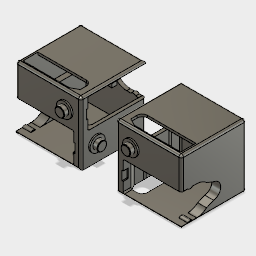
servo_assem_type2 (Autodesk Fusion 360 design; units mm, degrees)
Autodesk Fusion 360 part; units mm, degrees
sketch "スケッチ1" plane through (0, 0, 0) normal (0, 1, 0) x (1, 0, 0)
  line L0 (12.9, -12.9) -> (-12.9, -12.9)
  line L1 (-12.9, -12.9) -> (-12.9, 12.9)
  line L2 (-12.9, 12.9) -> (12.9, 12.9)
  line L3 (12.9, 12.9) -> (12.9, -12.9)
  line L4 (12.9, -12.9) -> (-12.9, 12.9) construction
  line L5 (-12.9, -12.9) -> (12.9, 12.9) construction
  line L6 (12.9, 12.9) -> (11.6, 12.9)
  line L7 (11.6, 12.9) -> (11.6, 11.4)
  line L8 (11.6, 11.4) -> (12.9, 11.4)
  line L9 (12.9, 11.4) -> (12.9, 12.9)
  line L10 (11.6, 11.4) -> (5.6, 11.4)
  line L11 (5.6, 11.4) -> (5.6, -9.858)
  line L12 (5.6, -9.858) -> (11.6, -9.858)
  line L13 (11.6, -9.858) -> (11.6, 11.4)
  line L14 (11.6, -9.858) -> (10.1, -9.858)
  line L15 (11.6, -9.858) -> (13.1, -9.858) construction
  line L16 (10.1, -9.858) -> (11.6, -7.0369)
  line L17 (10.1, -9.858) -> (13.2951, -9.858) construction
  dimension "d1" = 25.8
  dimension "d2" = 25.8
  dimension "d10" = 1.5
  dimension "d11" = 1.3
  dimension "d12" = 6
  dimension "d13" = 21.258
  dimension "d14" = 180
  dimension "d15" = 1.5
  dimension "d16" = 62
  constraint perpendicular L0 L1
  constraint parallel L0 L2
  constraint parallel L1 L3
  constraint horizontal L0
  constraint coincident L4
  constraint coincident L5
  constraint horizontal L6
  constraint vertical L7
  constraint horizontal L8
  constraint vertical L9
  constraint horizontal L10
  constraint vertical L11
  constraint horizontal L12
  constraint vertical L13
  constraint horizontal L15
  constraint coincident L13
  constraint horizontal L17
  measures "d14" angle of L14 L15
  measures "d16" angle of L16 L17
extrude "押し出し1" add sketch "スケッチ1" along normal blind 0.95 contours L10 L11 L12 L13 L16 | L0 L1 L2 L3 L7 L8 | L2 L3 L6 L7 L8 L9 | L12 L13 L14 L16 makes body 1
extrude "押し出し2" cut sketch "スケッチ1" along normal blind 5 contours L10 L11 L12 L13 L16 bodies 1
fillet "フィレット1" radius 2 1 edges at (5.6, 0.475, 9.858) on bodies 1
ref_plane "作業平面1" through (12.9, 0.475, 0) normal (1, 0, 0) x (0, 0, -1)
ref_plane "作業平面2" through (0, 0.475, 12.9) normal (0, 0, 1) x (1, 0, 0)
ref_plane "作業平面3" through (-12.9, 0.475, 0) normal (-1, 0, 0) x (0, 0, 1)
ref_plane "作業平面4" through (0, 0.475, -12.9) normal (0, 0, -1) x (-1, 0, 0)
ref_plane "作業平面5" through (0, 25.2, 0) normal (0, -1, 0) x (-1, 0, 0)
sketch "スケッチ2" plane through (-12.9, 0.475, 0) normal (-1, 0, 0) x (0, 0, -1)
  line L0 (-12.9, 0.475) -> (12.9, 0.475)
  line L1 (12.9, 0.475) -> (12.9, -24.725)
  line L2 (12.9, -24.725) -> (-12.9, -24.725)
  line L3 (-12.9, -24.725) -> (-12.9, 0.475)
  line L4 (-12.9, 0.475) -> (-6.8, 0.475)
  line L5 (-6.8, 0.475) -> (-6.8, -6.325) construction
  line L6 (-6.8, -6.325) -> (-12.9, -6.325) construction
  line L7 (-12.9, -6.325) -> (-12.9, 0.475)
  line L8 (-6.8, -6.325) -> (-0.431, -6.325)
  circle A0 centre (-0.431, -6.325) radius 3.1815
  circle A1 centre (-6.8, -6.325) radius 5.85
  line L9 (-0.431, -6.325) -> (-0.0874, -9.4879) construction
  line L10 (-0.431, -6.325) -> (2.7505, -6.325) construction
  line L11 (-0.431, -6.325) -> (-0.0874, -3.1621) construction
  line L12 (-6.8, -6.325) -> (-2.878, -10.6656) construction
  line L13 (-6.8, -6.325) -> (-0.95, -6.325) construction
  line L14 (-6.8, -6.325) -> (-2.878, -1.9844) construction
  line L15 (-0.0874, -9.4879) -> (-2.878, -10.6656)
  line L16 (-0.0874, -3.1621) -> (-2.878, -1.9844)
  line L17 (-6.8, -6.325) -> (-6.8, -12.175) construction
  line L18 (-6.8, -12.175) -> (-12.9, -12.175)
  line L19 (-6.8, -0.475) -> (-12.9, -0.475)
  line L20 (-12.9, -12.175) -> (-9.4, -12.175)
  line L21 (-12.9, -0.475) -> (-9.4, -0.475)
  line L22 (-9.4, -12.175) -> (-9.4, -12.975) construction
  line L23 (-9.4, -12.175) -> (-8.6, -12.175) construction
  line L24 (-9.4, -0.475) -> (-9.4, 0.325) construction
  line L25 (-9.4, -0.475) -> (-10.2, -0.475) construction
  circle A2 centre (-9.4, -12.975) radius 1.25
  circle A3 centre (-9.4, 0.325) radius 1.25
  line L26 (-12.9, -12.175) -> (-2.9, -12.175) construction
  line L27 (-2.9, -12.175) -> (12.9, -12.175)
  line L28 (-12.9, -12.175) -> (-2.9, -12.175)
  line L29 (-2.9, -12.175) -> (-2.9, -10.6853)
  line L30 (-2.9, -12.175) -> (-4.3897, -12.175) construction
  dimension "d20" = 25.8
  dimension "d21" = 25.2
  dimension "d22" = 6.1
  dimension "d23" = 6.8
  dimension "d24" = 6.369
  dimension "d25" = 6.363
  dimension "d26" = 11.7
  dimension "d27" = 83.8
  dimension "d28" = 83.8
  dimension "d29" = 47.9
  dimension "d30" = 47.9
  dimension "d31" = 3.5
  dimension "d32" = 3.5
  dimension "d33" = 90
  dimension "d34" = 0.8
  dimension "d35" = 90
  dimension "d36" = 0.8
  dimension "d37" = 2.5
  dimension "d38" = 2.5
  dimension "d39" = 10
  dimension "d40" = 10
  dimension "d41" = 90
  constraint horizontal L0
  constraint vertical L1
  constraint horizontal L2
  constraint vertical L3
  constraint horizontal L4
  constraint vertical L5
  constraint horizontal L6
  constraint vertical L7
  constraint coincident A0
  constraint horizontal L10
  constraint coincident A1
  constraint horizontal L13
  constraint perpendicular L13 L17
  constraint coincident L3
  constraint tangent A1 L18
  constraint coincident L5
  constraint horizontal L23
  constraint horizontal L25
  constraint coincident L1
  constraint perpendicular L1 L27
  constraint perpendicular L28 L29
  constraint horizontal L30
  measures "d25" diameter of A0
  measures "d26" diameter of A1
  measures "d27" angle of L9 L10
  measures "d28" angle of L10 L11
  measures "d29" angle of L12 L13
  measures "d30" angle of L13 L14
  measures "d33" angle of L22 L23
  measures "d35" angle of L24 L25
  measures "d37" diameter of A2
  measures "d38" diameter of A3
  measures "d41" angle of L29 L30
extrude "押し出し3" add sketch "スケッチ2" against normal blind 1.5 separate body contours L1 L2 L3 L18 L20 A2 L27 L28 | A1 L28 L29 | L18 L20 A2 L28 | L18 L20 A2 L28 makes body 2
extrude "押し出し4" add sketch "スケッチ2" against normal blind 3.5 contours L0 L1 L4 A0 A1 L15 L16 L19 A3 L27 L29 | L0 L4 L19 L21 A3 | L19 L21 A3 bodies 2
sketch "スケッチ4" plane through (0, 0.475, 12.9) normal (0, 0, 1) x (1, 0, 0)
  line L0 (-12.9, -0.475) -> (-12.9, 24.725)
  line L1 (-12.9, 24.725) -> (12.9, 24.725)
  line L2 (12.9, 24.725) -> (12.9, -0.475)
  line L3 (12.9, -0.475) -> (-12.9, -0.475)
  line L4 (-12.9, 24.725) -> (-12.9, -0.475)
  line L5 (-12.9, -0.475) -> (-12.9, 12.125)
  line L6 (-12.9, 12.125) -> (10.1, 12.125)
  line L7 (10.1, 12.125) -> (10.1, -0.475)
  line L8 (10.1, -0.475) -> (-12.9, -0.475)
  line L9 (12.9, 24.725) -> (6.8, 24.725)
  line L10 (6.8, 24.725) -> (6.8, 17.925) construction
  line L11 (6.8, 17.925) -> (12.9, 17.925) construction
  line L12 (12.9, 17.925) -> (12.9, 24.725)
  circle A0 centre (6.8, 17.925) radius 1.9
  circle A1 centre (6.8, 17.925) radius 3
  line L13 (10.1, -0.475) -> (10.1, 4.525)
  line L14 (10.1, -0.475) -> (5.1, -0.475) construction
  line L15 (10.1, 4.525) -> (10.6, 4.525)
  line L16 (10.6, 4.525) -> (10.6, 8.125)
  line L17 (10.6, 8.125) -> (10.1, 8.125)
  line L18 (10.1, 8.125) -> (10.1, 4.525)
  line L19 (10.1, 8.125) -> (10.1, 12.125)
  line L20 (10.1, 12.125) -> (12.9, 12.125)
  dimension "d68" = 23
  dimension "d69" = 6.8
  dimension "d70" = 6.1
  dimension "d71" = 3.8
  dimension "d72" = 6
  dimension "d73" = 90
  dimension "d74" = 5
  dimension "d75" = 3.6
  dimension "d76" = 0.5
  dimension "d102" = 12.6
  constraint perpendicular L0 L1
  constraint parallel L0 L2
  constraint parallel L1 L3
  constraint parallel L0 L4
  constraint perpendicular L5 L6
  constraint parallel L5 L7
  constraint parallel L6 L8
  constraint coincident L4
  constraint horizontal L9
  constraint vertical L10
  constraint horizontal L11
  constraint vertical L12
  constraint concentric A0 A1
  constraint horizontal L14
  constraint horizontal L15
  constraint vertical L16
  constraint horizontal L17
  constraint vertical L18
  constraint coincident L2
  constraint perpendicular L2 L20
  measures "d71" diameter of A0
  measures "d72" diameter of A1
  measures "d73" angle of L13 L14
  measures "d102" distance of L1 L6
extrude "押し出し10" add sketch "スケッチ4" against normal blind 1.3 separate body contours L0 L1 L2 L4 L6 L9 L12 L20 | A0 | A1 makes body 3
extrude "押し出し11" add sketch "スケッチ4" against normal blind 3 contours L2 L3 L7 L13 L15 L16 L17 L19 L20 bodies 3
extrude "押し出し12" add sketch "スケッチ4" along normal blind 0.6 contours A1 bodies 3
extrude "押し出し13" add sketch "スケッチ4" along normal blind 2.4 contours A0 bodies 3
sketch "スケッチ7" plane through (0, 25.2, 0) normal (0, 1, 0) x (-1, 0, 0)
  line L0 (12.9, 12.9) -> (-12.9, 12.9)
  line L1 (-12.9, 12.9) -> (-12.9, 11.6)
  line L2 (-12.9, 11.6) -> (12.9, 11.6)
  line L3 (12.9, 11.6) -> (12.9, 12.9)
  line L4 (-10.1, 11.6) -> (12.9, 11.6)
  line L5 (11.4006, 11.6) -> (7.1826, 11.6)
  line L6 (11.4, -12.9) -> (11.4, 12.9)
  line L7 (7.1826, 11.6) -> (7.1826, 12.75)
  line L8 (7.1826, 12.75) -> (-2.8174, 12.75)
  circle A0 centre (-2.8174, 12.75) radius 1.25
  circle A1 centre (7.1826, 12.75) radius 1.25
  dimension "d112" = 4.218
  dimension "d113" = 1.15
  dimension "d114" = 10
  dimension "d115" = 2.5
  dimension "d116" = 2.5
  constraint coincident L2
  constraint perpendicular L5 L6
  measures "d115" diameter of A0
  measures "d116" diameter of A1
extrude "押し出し20" add sketch "スケッチ7" against normal blind 12.6 contours L2 L4 L5 A1 | L2 L4 A0 bodies 3
copy_body "CopyPasteBodies2" bodies 3 makes body 4
move_body "ボディを移動2" bodies 4 to x (0, 0, 1) y (0, -1, 0) z (1, 0, 0) at (0, 25.2, 0)
copy_body "CopyPasteBodies3" bodies 1 makes body 5
move_body "ボディを移動3" bodies 5 to x (-1, 0, 0) y (0, 1, 0) z (0, 0, -1) at (0, 24.25, 0)
copy_body "CopyPasteBodies4" bodies 2 makes body 6
move_body "ボディを移動4" bodies 6 to x (0, 0, 1) y (0, -1, 0) z (1, 0, 0) at (0, 25.2, 0)
combine "結合1" operation add target body 1 tool bodies 2 3 4 5 6
chamfer "面取り1" distance 0.2 angle 45 2 edges at (5.0286, 17.7129, 15.3) (15.3, 7.4871, 5.0286) on bodies 1
fillet "フィレット2" radius 0.9 11 edges at (12.9, 25.2, 0) (0, 25.2, 12.9) (12.9, 12.6, 12.9) (0, 25.2, -12.9) (-12.9, 25.2, 0) (-12.9, 12.6, -12.9) (-12.9, 0, 0) (0, 0, -12.9) (0, 0, 12.9) (-12.9, 18.9, 12.9) (12.9, 6.3, -12.9) on bodies 1
fillet "フィレット6" radius 0.5 1 edges at (11.6, 6.275, -11.4) on bodies 1
sketch "スケッチ5" plane through (0, 25.2, 0) normal (0, 1, 0) x (-1, 0, 0)
  arc A0 (5.6, -7.858) -> (6.3263, -9.4) centre (7.6, -7.858) ccw
  line L0 (5.6, -7.858) -> (5.6, 11.4)
  line L1 (5.6, 11.4) -> (11.4, 11.4)
  line L2 (11.4, 11.4) -> (11.4, -7.4131)
  line L3 (11.4, -7.4131) -> (10.3435, -9.4)
  line L4 (10.3435, -9.4) -> (6.3263, -9.4)
  line L5 (-12, -12) -> (12, -12)
  line L6 (12, -12) -> (12, 12)
  line L7 (12, 12) -> (-12, 12)
  line L8 (-12, 12) -> (-12, -12)
  line L9 (5.6, 11.4) -> (11.4, 11.4)
  line L10 (11.4, 11.4) -> (11.4, -9.4)
  line L11 (11.4, -9.4) -> (5.6, -9.4)
  line L12 (5.6, -9.4) -> (5.6, 11.4)
  constraint vertical L10
  constraint horizontal L11
  constraint vertical L12
extrude "押し出し14" add sketch "スケッチ5" against normal blind 0.95 contours A0 L0 L1 L2 L3 L4 L9 L10 L11 L12 bodies 1
sketch "スケッチ6" plane through (0, 25.2, 0) normal (0, 1, 0) x (-1, 0, 0)
  line L0 (-12, -12) -> (12, -12)
  line L1 (12, -12) -> (12, 12)
  line L2 (12, 12) -> (-12, 12)
  line L3 (-12, 12) -> (-12, -12)
  line L4 (12.9, 12.9) -> (11.4, 12.9)
  line L5 (11.4, 12.9) -> (11.4, 11.6) construction
  line L6 (11.4, 11.6) -> (12.9, 11.6) construction
  line L7 (12.9, 11.6) -> (12.9, 12.9)
  line L8 (11.4, 11.6) -> (-9.858, 11.6)
  line L9 (-9.858, 11.6) -> (-9.858, 5.6)
  line L10 (-9.858, 5.6) -> (11.4, 5.6)
  line L11 (11.4, 5.6) -> (11.4, 11.6)
  line L12 (-9.858, 11.6) -> (-9.858, 10.1)
  line L13 (-9.858, 11.6) -> (-7.037, 11.6)
  line L14 (-7.037, 11.6) -> (-9.858, 10.1)
  dimension "d89" = 1.3
  dimension "d90" = 21.258
  dimension "d91" = 6
  dimension "d92" = 1.5
  dimension "d93" = 2.821
  constraint horizontal L4
  constraint vertical L5
  constraint horizontal L6
  constraint vertical L7
  constraint horizontal L8
  constraint vertical L9
  constraint horizontal L10
  constraint vertical L11
extrude "押し出し15" cut sketch "スケッチ6" against normal blind 5 contours L8 L9 L10 L11 L14 bodies 1
extrude "押し出し21" add 2 faces at (2.9279, 20.2, 11.5816) (-7.0721, 20.2, 11.5816) along direction (0, 1, 0) blind 5 on bodies 1 bodies 1
fillet "フィレット3" radius 2 1 edges at (9.858, 24.725, 5.6) on bodies 1
fillet "フィレット4" radius 0.5 1 edges at (-11.4, 18.925, 11.6) on bodies 1
extrude "押し出し16" add sketch "スケッチ1" along normal blind 12.6 contours L12 L13 L14 L16 bodies 1
extrude "押し出し17" add 1 faces at (10.6, 4.8333, 9.858) along direction (0, 0, 1) blind 1.042 on bodies 1 bodies 1
extrude "押し出し18" add sketch "スケッチ6" against normal blind 12.6 contours L8 L9 L12 L13 L14 bodies 1
extrude "押し出し19" add 1 faces at (9.858, 20.3667, 11.1) along direction (1, 0, 0) blind 1.042 on bodies 1 bodies 1
fillet "フィレット7" radius 0.5 4 edges at (10.1, 0.95, 11.379) (10.1, 12.6, 11.5) (11.5, 12.6, 10.1) (11.379, 24.25, 10.1) on bodies 1
ref_plane "作業平面6" through (19.9, 12.6, 0) normal (1, 0, 0) x (0, 0, -1)
mirror "ミラー1" about plane through (19.9, 12.6, 0) normal (1, 0, 0) of bodies 1 makes body 7
equation "d105 = 3.042 mm - 2 mm"
equation "d109 = 3.042 mm - 2 mm"
